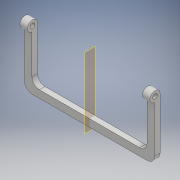
# Autodesk Inventor part: back_support
Saved by Autodesk Inventor 2018 (Build 220112000, 112)
## iProperties
Created: 2018-08-02
Part Number: back_support
Material: Generic
Document SubType Name: Modeling
Designer: Luke
Density: 1 g/cm^3
Appearance: Default
Author: Luke
Autodesk Inventor part; units mm, degrees
ref_plane "XZ Plane" through (0, 0, 0) normal (0, 1, 0) x (-1, 0, 0)
ref_plane "XY Plane" through (0, 0, 0) normal (0, 0, 1) x (1, 0, 0)
sketch "Sketch2" plane through (0, 0, 0) normal (0, 1, 0) x (-1, 0, 0)
  line L0 (35, -4) -> (35, 25)
  line L1 (35, 25) -> (31, 25)
  line L2 (31, 25) -> (31, 0)
  line L3 (31, 0) -> (-31, 0)
  line L4 (-31, 0) -> (-31, 25)
  line L5 (-31, 25) -> (-35, 25)
  line L6 (-35, 25) -> (-35, -4)
  line L7 (-35, -4) -> (35, -4)
  line L8 (0, -9.8) -> (0, 30.8) construction
  line L9 (-49, 0) -> (49, 0) construction
  point P0 (0, 0)
  dimension "d0" = 4
  dimension "d1" = 25
  dimension "d2" = 70
  dimension "d3" = 4
  constraints: 16 end point, 6 perpendicular, 2 point on line, 1 collinear, 1 vertical, 2 other
  measures "d0" distance between parallel lines of L2 L0
  measures "d1" distance of L1.end L2.end
  measures "d2" distance of L6.end L0.start
  measures "d3" distance between parallel lines of L7 L3
extrude "Extrusion1" add sketch "Sketch2" along normal blind 3
sketch "Sketch3" plane through (35, 0, 25) normal (1, 0, 0) x (0, 0, -1)
  line L0 (0, 0) -> (0, 3) construction
  line L1 (0, 0) -> (0, 3) construction
  line L2 (0, 0.25) -> (-2.7386, 0.25) construction
  circle A0 centre (-2.7386, 0.25) radius 1.25
  circle A1 centre (-2.7386, 0.25) radius 2.75
  line L3 (0, 0) -> (29, 0) construction
  line L4 (0, 3) -> (29, 3) construction
  line L5 (29, 3) -> (0, 3) construction
  line L6 (-2.7386, 3) -> (0, 3) construction
  line L7 (-2.7386, 3) -> (-2.7386, 0.25) construction
  line L8 (-2.7386, 3) -> (0, 3)
  line L9 (0, 0) -> (0, 3)
  point P0 (25, 0)
  dimension "d6" = 2.5
  dimension "d7" = 1.5
  constraints: 10 end point, 3 collinear, 2 centre point, 2 coincident, 2 point on circle, 1 horizontal, 1 perpendicular, 1 point on line, 1 tangent
  measures "d6" diameter of A0
  measures "d7" radial gap between concentric circles of A1 A0
extrude "Extrusion2" add sketch "Sketch3" against normal up to surface (4 mm away)
mirror "Mirror1" about plane through (0, 0, 0) normal (1, 0, 0) of "Extrusion2"
fillet "Fillet1" radius 4 4 edges at (-35, 1.5, -4) (-31, 1.5, 0) (31, 1.5, 0) (35, 1.5, -4)
equation "\"d3\" = d0"
body "Solid1"
